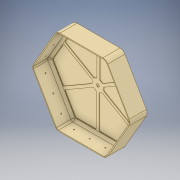
# Autodesk Inventor part: Base
Saved by Autodesk Inventor 2019 (Build 230136000, 136)
## iProperties
Created: 2021-07-14
Part Number: Base
Material: Generic
Document SubType Name: Modeling
Designer: Lix
Density: 1 g/cm^3
Appearance: Beige
Author: Lix
Autodesk Inventor part; units mm, degrees
sketch "Sketch1" plane through (0, 0, 0) normal (0, 0, 1) x (1, 0, 0)
  line L0 (43.3013, -75) -> (-43.3013, -75)
  line L1 (-43.3013, -75) -> (-86.6025, 0)
  line L2 (-86.6025, 0) -> (-43.3013, 75)
  line L3 (-43.3013, 75) -> (43.3013, 75)
  line L4 (43.3013, 75) -> (86.6025, 0)
  line L5 (86.6025, 0) -> (43.3013, -75)
  point P0 (0, 0)
  point P1 (0, 0)
  point P2 (0, 0)
  dimension "d0" = 150
  constraints: 12 end point, 2 coincident, 1 horizontal, 13 other
  measures "d0" distance between parallel lines of L5 L2
extrude "Extrusion1" add sketch "Sketch1" along normal blind 30
shell "Shell1" thickness 1.5 removed faces 1 at (0, 0, 30) ; own thickness 1 on faces at (0, 0, 0)
sketch "Sketch2" plane through (-84.8705, 0, 30) normal (0.8660254, 0.5, 0) x (0, 0, -1)
  circle A0 centre (14.5, -69.8705) radius 1
  circle A1 centre (14.5, -15) radius 1
  line L0 (29, -84.8705) -> (0, -84.8705) projected
  line L1 (29, 0) -> (0, 0) projected
  circle A2 centre (14.5, -42.4352) radius 1
  line L2 (29, -84.8705) -> (29, 0) projected
  line L3 (29, 0) -> (0, 0) projected
  line L4 (0, -84.8705) -> (0, 0) projected
  line L5 (29, -84.8705) -> (0, -84.8705) projected
  line L6 (0, -84.8705) -> (0, 0) projected
  point P0 (30, -42.4352)
  point P1 (14.5, -84.8705)
  point P2 (0, -42.4352)
  dimension "d5" = 2
  dimension "d6" = 15
  dimension "d7" = 15
  constraints: 3 centre point, 3 vertical alignment, 2 equal radius, 2 midpoint, 1 horizontal alignment
  measures "d5" diameter of A0
  measures "d6" distance of A0.centre point (14.5, -84.87)
  measures "d7" distance from line of L1 A1.centre
ref_plane "Work Plane1" through (-21.6506, 37.5, 30) normal (0.8660254, 0.5, 0) x (0, 0, -1)
ref_plane "Work Plane2" through (-43.3013, 0, 0) normal (0, 1, 0) x (1, 0, 0)
ref_plane "Work Plane3" through (-21.6506, -37.5, 0) normal (-0.8660254, 0.5, 0) x (0, 0, 1)
sketch "Sketch4" plane through (-42.4352, -73.5, 1) normal (0, 0, 1) x (1, 0, 0)
  line L0 (84.8705, 0) -> (0, 0) projected
  line L1 (127.3057, 73.5) -> (84.8705, 0) projected
  line L2 (84.8705, 147) -> (127.3057, 73.5) projected
  line L3 (0, 147) -> (84.8705, 147) projected
  line L4 (-42.4352, 73.5) -> (0, 147) projected
  line L5 (0, 0) -> (-42.4352, 73.5) projected
  line L6 (-15.3853, 110.352) -> (2.8868, 142)
  line L7 (2.8868, 142) -> (40.5972, 142)
  line L8 (84.8705, 147) -> (0, 0) construction
  arc A0 (40.5972, 83.3296) -> (35.6774, 80.8709) centre (42.4352, 73.5) ccw
  line L9 (-15.3853, 110.352) -> (35.6774, 80.8709)
  line L10 (40.5972, 142) -> (40.5972, 83.3296)
  line L11 (-18.3897, 41.852) -> (-36.6617, 73.5)
  line L12 (-36.6617, 73.5) -> (-17.8065, 106.1582)
  line L13 (-17.8065, 106.1582) -> (33.0035, 76.823)
  arc A1 (33.0035, 76.823) -> (32.6729, 71.333) centre (42.4352, 73.5) ccw
  line L14 (-18.3897, 41.852) -> (32.6729, 71.333)
  line L15 (39.4308, 5) -> (2.8868, 5)
  line L16 (2.8868, 5) -> (-15.9685, 37.6582)
  line L17 (-15.9685, 37.6582) -> (34.8416, 66.9934)
  arc A2 (34.8416, 66.9934) -> (39.4308, 63.962) centre (42.4352, 73.5) ccw
  line L18 (39.4308, 5) -> (39.4308, 63.962)
  line L19 (100.2557, 36.648) -> (81.9837, 5)
  line L20 (81.9837, 5) -> (44.2733, 5)
  line L21 (44.2733, 5) -> (44.2733, 63.6704)
  arc A3 (44.2733, 63.6704) -> (49.1931, 66.1291) centre (42.4352, 73.5) ccw
  line L22 (100.2557, 36.648) -> (49.1931, 66.1291)
  line L23 (103.2602, 105.148) -> (121.5322, 73.5)
  line L24 (121.5322, 73.5) -> (102.677, 40.8418)
  line L25 (102.677, 40.8418) -> (51.867, 70.177)
  arc A4 (51.867, 70.177) -> (52.1976, 75.667) centre (42.4352, 73.5) ccw
  line L26 (103.2602, 105.148) -> (52.1976, 75.667)
  line L27 (45.4397, 142) -> (81.9837, 142)
  line L28 (81.9837, 142) -> (100.839, 109.3418)
  line L29 (100.839, 109.3418) -> (50.0289, 80.0066)
  arc A5 (50.0289, 80.0066) -> (45.4397, 83.038) centre (42.4352, 73.5) ccw
  line L30 (45.4397, 142) -> (45.4397, 83.038)
  circle A6 centre (42.4352, 73.5) radius 2.5
  dimension "d37" = 5
  dimension "d44" = 10
  dimension "d45" = 60
  dimension "d46" = 90
  dimension "d47" = 90
  dimension "d50" = 360
  dimension "d52" = 5.5
  dimension "d55" = 5
  constraints: 50 end point, 12 point on circle, 7 centre point, 4 coincident, 1 midpoint, 65 other
  measures "d37" distance between parallel lines of L3 L7
  measures "d44" radius of A0
  measures "d45" angle of L10 L9
  measures "d46" angle of L9 L6
  measures "d47" angle of L10 L7
  measures "d52" distance of L10.end L9.end
  measures "d55" diameter of A6
extrude "Extrusion5" cut sketch "Sketch4" against normal blind 0.75 contours L6 L7 L10 A0 L9 | L11 L12 L13 A1 L14 | L15 L16 L17 A2 L18 | L19 L20 L21 A3 L22 | L23 L24 L25 A4 L26 | L27 L28 L29 A5 L30 | A6
extrude "Extrusion2" cut sketch "Sketch2" against normal blind 1 contours A0 | A1 | A2
mirror "Mirror1" about plane through (-21.6506, 37.5, 30) normal (0.8660254, 0.5, 0) of "Extrusion2"
mirror "Mirror2" about plane through (-43.3013, 0, 0) normal (0, 1, 0) of "Extrusion2"
mirror "Mirror3" about plane through (-21.6506, -37.5, 0) normal (-0.8660254, 0.5, 0) of "Extrusion2", "Mirror2"
mirror "Mirror4" about plane through (-43.3013, 0, 0) normal (0, 1, 0) of "Extrusion2", "Mirror2", "Mirror3"
fillet "Fillet1" radius 4 12 edges at (0, -73.5, 1) (-63.6529, -36.75, 1) (63.6529, -36.75, 1) (63.6529, 36.75, 1) (0, 73.5, 1) (-63.6529, 36.75, 1) (-84.8705, 0, 15.5) (-42.4352, 73.5, 15.5) (42.4352, 73.5, 15.5) (84.8705, 0, 15.5) (42.4352, -73.5, 15.5) (-42.4352, -73.5, 15.5)
fillet "Fillet2" radius 10 6 edges at (86.6025, 0, 15) (43.3013, 75, 15) (-43.3013, 75, 15) (43.3013, -75, 15) (-86.6025, 0, 15) (-43.3013, -75, 15)
fillet "Fillet4" radius 2 30 edges at (-7.5937, -6.5066, 0.625) (-9.7624, -2.167, 0.625) (-9.4317, 3.323, 0.625) (-6.7579, 7.3709, 0.625) (-1.838, 9.8296, 0.625) (3.0045, 9.538, 0.625) (7.5937, 6.5066, 0.625) (9.7624, 2.167, 0.625) (9.4317, -3.323, 0.625) (6.7579, -7.3709, 0.625) (1.838, -9.8296, 0.625) (-3.0045, -9.538, 0.625) (-60.2418, 32.6582, 0.625) (-79.097, 0, 0.625) (-60.825, -31.648, 0.625) (-58.4037, -35.8418, 0.625) (-39.5485, -68.5, 0.625) (-3.0045, -68.5, 0.625) (1.838, -68.5, 0.625) (39.5485, -68.5, 0.625) (57.8205, -36.852, 0.625) (60.2418, -32.6582, 0.625) (79.097, 0, 0.625) (60.825, 31.648, 0.625) (58.4037, 35.8418, 0.625) (39.5485, 68.5, 0.625) (-1.838, 68.5, 0.625) (3.0045, 68.5, 0.625) (-39.5485, 68.5, 0.625) (-57.8205, 36.852, 0.625)
equation "\"d7\" = d6"
body "Solid1"
